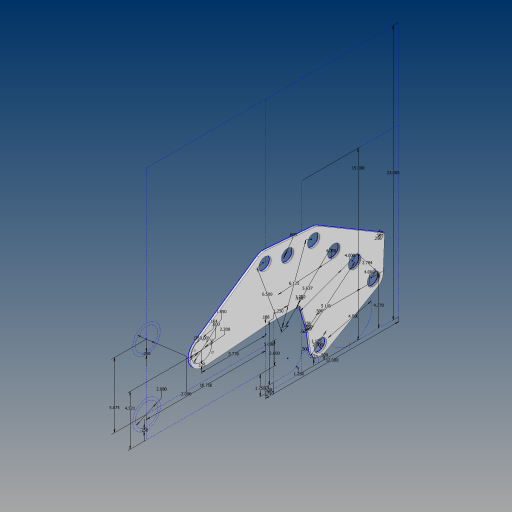
# Autodesk Inventor part: Intake Roller Plate
Saved by Autodesk Inventor 2024.3 (Build 283343000, 343)
## iProperties
Created: 2024-07-25
Part Number: Intake Roller Plate
Material: Aluminum 6061
Document SubType Name: Modeling
Designer: Kenji
Density: 2.7 g/cm^3
Appearance: Aluminum - Dark
Author: Kenji
Autodesk Inventor part; units mm, degrees
ref_plane "YZ Plane" through (0, 0, 0) normal (1, 0, 0) x (0, 1, 0)
ref_plane "XZ Plane" through (0, 0, 0) normal (0, 1, 0) x (-1, 0, 0)
ref_plane "XY Plane" through (0, 0, 0) normal (0, 0, 1) x (1, 0, 0)
sketch "Sketch1" plane through (0, 0, 0) normal (1, 0, 0) x (0, 1, 0)
  line L0 (127, 0) -> (127, -31.75) construction
  line L1 (95.25, -63.5) -> (31.75, -63.5) construction
  line L2 (0, -31.75) -> (0, 0) construction
  arc A0 (95.25, -63.5) -> (127, -31.75) centre (95.25, -31.75) ccw construction
  arc A1 (0, -31.75) -> (31.75, -63.5) centre (31.75, -31.75) ccw construction
  line L3 (0, 0) -> (0, 19.05) construction
  line L4 (0, 19.05) -> (-12.7, 19.05) construction
  line L5 (82.55, 19.05) -> (82.55, 292.1) construction
  circle A2 centre (82.55, 292.1) radius 25.4 construction
  circle A3 centre (82.55, 292.1) radius 31.75 construction
  circle A4 centre (231.775, 292.1) radius 25.4 construction
  circle A5 centre (231.775, 292.1) radius 31.75 construction
  line L6 (-12.7, 19.05) -> (82.55, 19.05) construction
  line L7 (127, 0) -> (0, 0) construction
  line L8 (-12.7, 19.05) -> (-12.7, -285.75) construction
  circle A6 centre (38.1, -173.5122) radius 50.8 construction
  circle A7 centre (95.7575, -223.3324) radius 25.4 construction
  circle A8 centre (95.7575, -223.3324) radius 14.2875
  circle A9 centre (151.5813, -179.9391) radius 25.4 construction
  circle A10 centre (151.5813, -179.9391) radius 14.2875
  circle A11 centre (241.0272, -86.0847) radius 22.225 construction
  circle A12 centre (241.0272, -86.0847) radius 25.4 construction
  circle A13 centre (241.0272, -86.0847) radius 14.2875
  line L9 (82.55, 19.05) -> (127, 19.05) construction
  line L10 (127, 19.05) -> (127, 0) construction
  circle A14 centre (151.5813, -179.9391) radius 22.225 construction
  circle A15 centre (95.7575, -223.3324) radius 22.225 construction
  circle A16 centre (25.4, -101.6) radius 25.4 construction
  circle A17 centre (25.4, -101.6) radius 22.225 construction
  line L11 (25.4, -76.2) -> (25.4, -63.5) construction
  circle A18 centre (196.9415, -132.5571) radius 25.4 construction
  circle A19 centre (196.9415, -132.5571) radius 22.225 construction
  circle A20 centre (196.9415, -132.5571) radius 14.2875
  line L12 (0, -101.6) -> (-12.7, -101.6) construction
  circle A21 centre (68.9231, -79.375) radius 6.477 construction
  circle A22 centre (25.4, -101.6) radius 14.2875
  circle A23 centre (68.9231, -79.375) radius 3.2512
  circle A24 centre (86.0308, -147.7557) radius 50.8 construction
  circle A25 centre (128.4053, -107.3491) radius 50.8 construction
  circle A26 centre (107.4528, -121.7556) radius 50.8 construction
  circle A27 centre (172.6999, -60.316) radius 50.8 construction
  circle A28 centre (170.5551, -242.3062) radius 3.2512
  line L13 (127, 18.8609) -> (127, -51.915)
  line L14 (123.5762, -56.4949) -> (67.09, -73.1628)
  arc A29 (123.5762, -56.4949) -> (127, -51.915) centre (122.2248, -51.915) ccw
  circle A30 centre (241.0272, -26.5845) radius 25.4 construction
  circle A31 centre (241.0272, -26.5845) radius 14.2875
  circle A32 centre (241.0272, -26.5845) radius 22.225 construction
  line L15 (176.0843, -245.5809) -> (262.8818, -99.0283)
  line L16 (241.0272, -26.5845) -> (241.0272, -86.0847) construction
  line L17 (196.9415, -132.5571) -> (151.5813, -179.9391) construction
  line L18 (151.5813, -179.9391) -> (95.7575, -223.3324) construction
  line L19 (82.55, 19.05) -> (31.75, 19.05) construction
  line L20 (31.75, 19.05) -> (31.75, 292.1) construction
  line L21 (31.75, 292.1) -> (82.55, 292.1) construction
  arc A33 (262.8818, -99.0283) -> (266.3404, -88.1832) centre (241.0272, -86.0847) ccw
  circle A34 centre (177.8, 15.945) radius 50.8 construction
  circle A35 centre (250.2464, 25.1193) radius 14.2875
  circle A36 centre (250.2464, 25.1193) radius 22.225 construction
  line L22 (250.2464, 25.1193) -> (241.0272, -26.5845) construction
  circle A37 centre (241.0272, -26.5845) radius 7.62 construction
  circle A38 centre (250.2464, 25.1193) radius 25.4 construction
  line L23 (266.3404, -88.1832) -> (275.5596, 23.0208)
  line L24 (-12.7, -285.75) -> (571.5, -285.75) construction
  line L25 (571.5, -285.75) -> (571.5, 292.1) construction
  line L26 (31.75, 292.1) -> (571.5, 292.1) construction
  line L27 (127, 19.05) -> (571.5, 19.05) construction
  circle A39 centre (146.5717, 165.8007) radius 7.62 construction
  circle A40 centre (146.5717, 165.8007) radius 23.495 construction
  circle A41 centre (170.0667, 165.8007) radius 2.0828
  circle A42 centre (146.5717, 165.8007) radius 27.94 construction
  line L28 (115.5542, 163.3402) -> (126.985, 19.2385)
  arc A43 (127, 18.8609) -> (126.985, 19.2385) centre (122.2248, 18.8609) ccw
  arc A44 (275.5596, 23.0208) -> (271.1757, 39.5112) centre (250.2464, 25.1193) ccw
  circle A45 centre (146.5717, 165.8007) radius 31.115 construction
  line L29 (271.1757, 39.5112) -> (172.21, 183.4307)
  arc A46 (172.21, 183.4307) -> (115.5542, 163.3402) centre (146.5717, 165.8007) ccw
  circle A47 centre (158.3192, 186.1479) radius 2.0828
  circle A48 centre (134.8242, 186.1479) radius 2.0828
  circle A49 centre (123.0767, 165.8007) radius 2.0828
  circle A50 centre (134.8242, 145.4534) radius 2.0828
  circle A51 centre (158.3192, 145.4534) radius 2.0828
  line L30 (-12.7, -63.5) -> (368.3, -63.5) construction
  arc A52 (76.5152, -234.4538) -> (94.8208, -245.5376) centre (95.7575, -223.3324) ccw
  circle A53 centre (170.5551, -242.3062) radius 6.4262 construction
  line L31 (170.5551, -248.7324) -> (94.8208, -245.5376)
  arc A54 (170.5551, -248.7324) -> (176.0843, -245.5809) centre (170.5551, -242.3062) ccw
  line L32 (368.3, -63.5) -> (368.3, -285.75) construction
  line L33 (6.1577, -112.7214) -> (76.5152, -234.4538)
  arc A55 (22.2666, -79.597) -> (6.1577, -112.7214) centre (25.4, -101.6) ccw
  line L34 (66.4118, -73.3103) -> (22.2666, -79.597)
  arc A56 (66.4118, -73.3103) -> (67.09, -73.1628) centre (65.7386, -68.5828) ccw
  line L35 (8.1576, -115.6232) -> (81.7343, -206.09) construction
  circle A57 centre (68.9231, -79.375) radius 6.35 construction
  point P0 (-12.7, -173.5122)
  point P1 (176.9813, -179.9391)
  point P2 (127, -55.4847)
  point P3 (66.7563, -73.2613)
  point P4 (104.775, 19.05)
  point P5 (176.9813, -242.3062)
  point P6 (95.7575, -248.7324)
  dimension "d58" = 101.6
  dimension "d191" = 12.954
  dimension "d284" = 46.99
  dimension "d2" = 31.75
  dimension "d3" = 19.05
  dimension "d4" = 12.7
  dimension "d7" = 273.05
  dimension "d8" = 50.8
  dimension "d9" = 6.35
  dimension "d10" = 50.8
  dimension "d11" = 6.35
  dimension "d12" = 149.225
  dimension "d14" = 127
  dimension "d16" = 304.8
  dimension "d175" = 31.75
  dimension "d180" = 50.8
  dimension "d181" = 3.175
  dimension "d182" = 12.7
  dimension "d187" = 31.75
  dimension "d189" = 12.7
  dimension "d192" = 28.575
  dimension "d201" = 6.5024
  dimension "d207" = 101.6
  dimension "d208" = 101.6
  dimension "d210" = 130.175
  dimension "d214" = 15.875
  dimension "d216" = 101.6
  dimension "d218" = 6.5024
  dimension "d219" = 108.4575
  dimension "d220" = 143.1895
  dimension "d221" = 155.574
  dimension "d222" = 70.7056
  dimension "d224" = 4.7752
  dimension "d236" = 50.8
  dimension "d237" = 44.45
  dimension "d261" = 165.1
  dimension "d267" = 15.24
  dimension "d271" = 584.2
  dimension "d283" = 15.24
  dimension "d285" = 4.1656
  dimension "d290" = 55.88
  dimension "d291" = 4.7752
  dimension "d292" = 3.175
  dimension "d313" = 146.7507
  dimension "d318" = 114.8217
  dimension "d321" = 360
  dimension "d323" = 381
  dimension "d328" = 3.175
  dimension "d335" = 4.7752
  dimension "d336" = 12.7
  constraints: 73 end point, 52 centre point, 37 point on circle, 33 tangent, 18 point on line, 17 coincident, 17 equal radius, 10 perpendicular, 9 horizontal alignment, 8 concentric, 5 vertical, 5 vertical alignment, 4 horizontal, 3 parallel, 1 collinear, 1 midpoint, 40 other
  measures "d2" radius of A0
  measures "d3" distance of L2.end L3.end
  measures "d4" distance of L3.end L4.end
  measures "d7" distance of L5.start L5.end
  measures "d8" diameter of A2
  measures "d9" radial gap between concentric circles of A2 A3
  measures "d10" diameter of A4
  measures "d11" radial gap between concentric circles of A4 A5
  measures "d12" distance of L21.end A4.centre
  measures "d14" distance of L0.start L2.end
  measures "d16" distance of L4.end L8.end
  measures "d175" radius of A1
  measures "d180" diameter of A16
  measures "d181" radial gap between concentric circles of A16 A17
  measures "d182" distance of L11.start L11.end
  measures "d187" distance of L0.start L0.end
  measures "d189" distance of L12.start L12.end
  measures "d192" diameter of A22
  measures "d201" diameter of A23
  measures "d207" diameter of A24
  measures "d208" diameter of A25
  measures "d210" distance of point (68.923, -79.375) A14.centre
  measures "d214" distance from line of L1 point (68.923, -79.375)
  measures "d216" diameter of A27
  measures "d218" diameter of A28
  measures "d219" distance from line of L8 point (95.757, -223.332)
  measures "d220" distance of A0.centre A18.centre
  measures "d221" distance of A0.centre A11.centre
  measures "d222" distance of point (95.757, -223.332) A14.centre
  measures "d224" radius of A29
  measures "d236" distance of L5.start L19.end
  measures "d237" distance of L4.end L19.end
  measures "d261" distance of A0.centre A36.centre
  measures "d267" diameter of A37
  measures "d271" distance of L8.end L24.end
  measures "d283" diameter of A39
  measures "d285" diameter of A41
  measures "d290" diameter of A42
  measures "d291" radius of A43
  measures "d313" distance from line of L9 point (146.572, 165.801)
  measures "d318" distance from line of L20 point (146.572, 165.801)
  measures "d323" distance of L30.start L30.end
  measures "d328" radial gap between concentric circles of A28 A53
  measures "d335" radius of A56
  measures "d336" diameter of A57
extrude "Extrusion4" add sketch "Sketch1" along normal blind 4.7625
body "Solid3"
